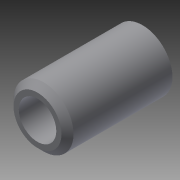
# Autodesk Inventor part: Spacer
Saved by Autodesk Inventor 2015 SP1 (Build 190203100, 203)
## iProperties
Created: 2016-04-11
Part Number: Spacer
Material: Generic
Document SubType Name: Modeling
Designer: jonesdm
Density: 1 g/cm^3
Appearance: Default
Author: jonesdm
Quantity: 1
Autodesk Inventor part; units mm, degrees
ref_plane "YZ Plane" through (0, 0, 0) normal (1, 0, 0) x (0, 1, 0)
ref_plane "XZ Plane" through (0, 0, 0) normal (0, 1, 0) x (-1, 0, 0)
ref_plane "XY Plane" through (0, 0, 0) normal (0, 0, 1) x (1, 0, 0)
sketch "Sketch1" plane through (0, 0, 0) normal (0, 0, 1) x (1, 0, 0)
  circle A0 centre (0, 0) radius 12.7
  circle A1 centre (0, 0) radius 7.9375
  dimension "d0" = 25.4
  dimension "d2" = 15.875
  constraints: 2 centre point, 2 coincident
  measures "d0" diameter of A0
  measures "d2" diameter of A1
extrude "Extrusion1" add sketch "Sketch1" along normal blind 44.45
chamfer "Chamfer1" distance 2.54 angle 45 1 edges at (-12.7, 0, 44.45)
body "Solid1"
